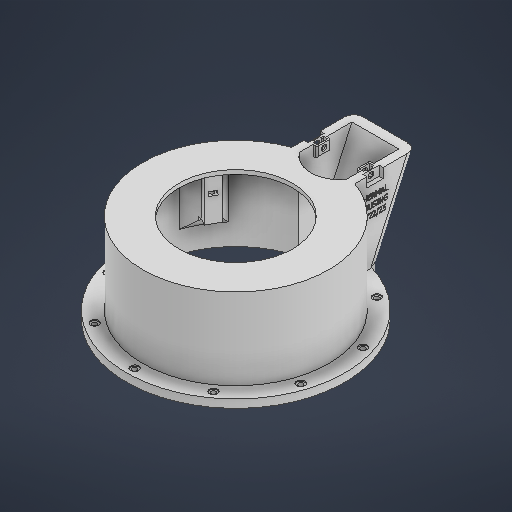
# Autodesk Inventor part: Thermal Housing
Saved by Autodesk Inventor 2026.2 (Build 302298000, 298)
## iProperties
Created: 2025-12-15
Part Number: Thermal Housing
Material: Generic
Document SubType Name: Modeling
Designer: mayhe
Density: 1 g/cm^3
Appearance: Default
Author: mayhe
Autodesk Inventor part; units mm, degrees
ref_plane "YZ Plane" through (0, 0, 0) normal (1, 0, 0) x (0, 1, 0)
ref_plane "XZ Plane" through (0, 0, 0) normal (0, 1, 0) x (-1, 0, 0)
ref_plane "XY Plane" through (0, 0, 0) normal (0, 0, 1) x (1, 0, 0)
sketch "Sketch1" plane through (0, 0, 0) normal (0, 1, 0) x (-1, 0, 0)
  circle A0 centre (0, 0) radius 135
  circle A1 centre (0, 0) radius 110.125
  circle A2 centre (0, 0) radius 115
  line L0 (39, -133.175) -> (-39, -133.175)
  line L1 (-39, -133.175) -> (-39, -87.525)
  line L2 (-39, -87.525) -> (39, -87.525)
  line L3 (39, -87.525) -> (39, -130.675)
  line L4 (39, -130.675) -> (39, -133.175)
  point P0 (0, -135)
  point P1 (39, -129.244)
  point P2 (-39, -129.244)
  point P3 (39, -130.675)
  point P4 (39, -102.9879)
  point P5 (39, -108.185)
  point P6 (-39, -108.185)
  point P7 (-39, -102.9879)
  dimension "d0" = 270
  dimension "d1" = 220.25
  dimension "d10" = 4.875
  dimension "d17" = 78
  dimension "d38" = 133.175
  dimension "d106" = 39
  dimension "d107" = 78
  constraints: 10 end point, 2 centre point, 2 coincident, 2 parallel, 1 horizontal, 1 perpendicular, 3 other
  measures "d1" diameter of A1
  measures "d10" radial gap between concentric circles of A1 A2
  measures "d17" distance of L1.end L2.end
  measures "d38" distance from line of A1.centre L0
  measures "d106" distance from line of point (0, 0) L1
  measures "d107" distance of L0.start L0.end
extrude "Cylinder Base" add sketch "Sketch1" along normal blind 10 contours A0 L3 A2 L1 | L1 A2 L3 A0 L0 | A0 L0 L1 | L3 L4 L0 A0 | L1 A1 L3 A2 | A2 L3 A1 L1
extrude "Cylinder Walls" add sketch "Sketch1" along normal blind 110.5 contours A2 L3 A1 L1 picked at (82.5972, -75.0251)
sketch "Sketch4" plane through (0, 110.5, 0) normal (0, 1, 0) x (1, 0, 0)
  circle A0 centre (0, 0) radius 110.125
  circle A1 centre (0, 0) radius 70.375
  dimension "d27" = 140.75
  constraints: 2 centre point, 2 coincident
  measures "d27" diameter of A1
extrude "Cylinder Top" add sketch "Sketch4" against normal blind 5
sketch "Sketch5" plane through (0, 110.5, 0) normal (0, 1, 0) x (1, 0, 0)
  line L0 (39, 108.185) -> (39, 185)
  line L1 (39, 185) -> (-39, 185)
  line L2 (-39, 185) -> (-39, 108.185)
  line L3 (-29, 172.6754) -> (29, 172.6754)
  line L4 (29, 172.6754) -> (29, 117.6754)
  line L5 (29, 117.6754) -> (-39, 117.6754)
  line L6 (-29, 117.6754) -> (-29, 172.6754)
  line L7 (-29, 172.6754) -> (29, 117.6754) construction
  line L8 (29, 172.6754) -> (-29, 117.6754) construction
  arc A0 (-29, 117.6754) -> (29, 117.6754) centre (0, 128.2867) ccw
  line L9 (39, 102.9879) -> (39, 108.185) projected
  line L10 (39, 108.185) -> (39, 102.9879)
  line L11 (-39, 108.185) -> (-39, 102.9879) projected
  line L12 (-39, 102.9879) -> (-39, 108.185)
  arc A1 (39, 102.9879) -> (-39, 102.9879) centre (0, 0) ccw projected
  line L13 (-39, 104.6754) -> (-39, 94.6754)
  line L14 (-39, 94.6754) -> (39, 94.6754)
  line L15 (39, 94.6754) -> (39, 102.9879)
  line L16 (29, 117.6754) -> (39, 117.6754)
  line L17 (-33.65, 177.3254) -> (33.65, 177.3254)
  line L18 (33.65, 177.3254) -> (33.65, 116.8811)
  arc A2 (-33.65, 116.8811) -> (33.65, 116.8811) centre (0, 128.2867) ccw
  line L19 (-33.65, 116.8811) -> (-33.65, 177.3254)
  line L20 (-29, 117.6754) -> (-29, 107.7584)
  line L21 (29, 117.6754) -> (29, 107.7584)
  point P0 (0, 113.425)
  point P1 (0, 145.1754)
  point P2 (23.0117, 107.6939)
  point P3 (-23.0117, 107.6939)
  point P4 (-39, 102.9879)
  point P5 (-39, 102.9879)
  point P6 (29, 106.238)
  point P7 (29, 106.4999)
  point P8 (-11.5192, 94.6754)
  point P9 (11.5192, 94.6754)
  point P10 (-33.65, 117.6754)
  point P11 (33.65, 117.6754)
  point P12 (-29, 106.238)
  point P13 (-28.0594, 106.4903)
  point P14 (28.0594, 106.4903)
  dimension "d33" = 78
  dimension "d36" = 55
  dimension "d72" = 185
  dimension "d115" = 10
  dimension "d132" = 78
  dimension "d133" = 10
  dimension "d134" = 23
  dimension "d135" = 4.65
  dimension "d150" = 10
  constraints: 40 end point, 7 point on circle, 4 point on line, 2 centre point, 2 midpoint, 2 parallel, 2 vertical, 1 perpendicular, 3 other
  measures "d33" distance between parallel lines of L2 L0
  measures "d36" distance of L3.end L4.end
  measures "d72" distance from line of point (0, 0) L1
  measures "d115" distance between parallel lines of L4 L0
  measures "d132" distance of L14.end L13.end
  measures "d133" distance of L13.end L13.start
  measures "d134" distance between parallel lines of L14 L5
  measures "d135" distance between parallel lines of L6 L19
  measures "d150" distance between parallel lines of L6 L2
sketch "Sketch6" plane through (0, 0, 0) normal (1, 0, 0) x (0, 1, 0)
  line L0 (110.5, -110.125) -> (110.5, -102.9879) projected
  line L1 (110.5, -178.433) -> (10, -133.175)
  line L2 (10, -133.175) -> (0, -133.175)
  point P0 (0, 0)
  point P1 (110.5, -108.185)
  dimension "d41" = 70.248
  constraints: 4 end point, 1 horizontal
  measures "d41" distance of point (110.5, -108.185) L1.start
sweep "Angled Camera Bracket" add profiles "Sketch5" path "Sketch6" keep normal constant yes path curves L1 L2 contours L9 A1 A2 L18 L16 L0 | L16 L18 L17 L19 L5 L2 L1 L0 | L18 A2 L21 L16 | L16 L4 L3 L6 L5 L19 L17 L18 | A1 A0 L21 A2 | L5 L19 A2 A1 L11 L2 | L20 A2 L19 L5 | A0 A1 A2 L20
extrude "Camera Clearance Cutout" cut sketch "Sketch5" against normal blind 25 contours A2 L14 A1 A0 | A1 A0 L21 A2 | A0 A1 L5 | A0 A1 | A2 L14 | A0 A1 A2 L20
sketch "Sketch7" plane through (0, 0, 0) normal (0, -1, 0) x (1, 0, 0)
  circle A0 centre (0, 0) radius 110.125
  constraints: 1 centre point, 1 coincident
extrude "Remove Excess from Sweep" cut sketch "Sketch7" against normal up to surface (105.5 mm away)
sketch "Sketch9" plane through (0, 0, 0) normal (1, 0, 0) x (0, 1, 0)
  point P0 (0, 0)
sketch "Sketch10" plane through (39, 110.5, -185) normal (0, -0.4106138, -0.9118093) x (-1, 0, 0)
  circle A0 centre (39, -58.2204) radius 3.5
  circle A1 centre (39, -44.2204) radius 3.5
  line L0 (78, 0) -> (78, -110.2204) projected
  line L1 (78, -110.2204) -> (0, -110.2204) projected
  point P0 (39, -176.7185)
  dimension "d61" = 7
  dimension "d63" = 7
  dimension "d64" = 14
  dimension "d108" = 39
  dimension "d168" = 52
  constraints: 2 centre point, 1 vertical alignment
  measures "d61" diameter of A0
  measures "d63" diameter of A1
  measures "d64" distance of A0.centre A1.centre
  measures "d108" distance from line of L0 A0.centre
  measures "d168" distance from line of L1 A0.centre
hole "Hole2" at (0, 70.1794, -166.8425) at (0, 57.4141, -161.0939) direction (0, 0.4106138, 0.9118093) diameter 7.25 depth 17.1 tip angle 118 counterbore diameter 12 counterbore depth 1.2
sketch "Sketch16" plane through (39, 0, -129.244) normal (1, 0, 0) x (0, 0, -1)
  line L0 (43.4315, 110.5) -> (-11.5685, 110.5) projected
  line L1 (-6.0589, 110.5) -> (13.9411, 110.5)
  line L2 (13.9411, 110.5) -> (13.9411, 98.5)
  line L3 (13.9411, 98.5) -> (-6.0589, 98.5)
  line L4 (-6.0589, 98.5) -> (-6.0589, 110.5)
  line L5 (-21.0589, 10) -> (-21.0589, 110.5) projected
  point P0 (-129.244, 0)
  point P1 (-22.7347, 10)
  dimension "d109" = 20
  dimension "d110" = 12
  dimension "d111" = 15
  constraints: 8 end point, 2 parallel, 1 horizontal, 1 perpendicular, 1 point on line, 1 other
  measures "d109" distance of L2.end L3.end
  measures "d110" distance of L1.end L2.end
extrude "Extrusion15" cut sketch "Sketch16" along normal through all both and the other way through all
sketch "Sketch17" plane through (39, 98.5, -123.185) normal (0, 1, 0) x (1, 0, 0)
  line L0 (-10, 0) -> (0, 0) projected
  line L1 (0, 20) -> (-10, 20) projected
  line L2 (-10, 0) -> (-5, 0)
  line L3 (-5, 0) -> (-5, 20)
  line L4 (-5, 20) -> (-7.675, 20)
  line L5 (-15, 1.5) -> (-10, 1.5)
  line L6 (-5, 3) -> (-5, 17)
  line L7 (-15, 18.5) -> (-15, 1.5)
  line L8 (-15, 1.5) -> (-5, 17) construction
  line L9 (-5, 3) -> (-15, 18.5) construction
  line L10 (-10, 1.5) -> (-10, 0)
  line L11 (-10, 0) -> (-10, 20) projected
  line L12 (-15, 18.5) -> (-10, 18.5)
  line L13 (-10, 18.5) -> (-10, 20)
  point P0 (-39, -123.185)
  point P1 (-5.35, 0)
  point P2 (-7.675, 20)
  dimension "d116" = 14
  dimension "d162" = 17
  dimension "d163" = 1.5
  constraints: 22 end point, 3 parallel, 3 perpendicular, 2 horizontal, 2 point on line, 1 collinear, 1 midpoint
  measures "d116" distance of L6.end L6.start
  measures "d162" distance of L7.start L5.start
  measures "d163" distance between parallel lines of L0 L5
extrude "Extrusion16" add sketch "Sketch17" along normal blind 12 and the other way blind 1
sketch "Sketch18" plane through (0, 110.5, 0) normal (0, 1, 0) x (1, 0, 0)
  line L0 (26, 126.685) -> (31.15, 126.685)
  line L1 (31.15, 126.685) -> (31.15, 139.685)
  line L2 (31.15, 139.685) -> (26, 139.685)
  line L3 (26, 139.685) -> (26, 126.685)
  line L4 (26, 126.685) -> (31.15, 139.685) construction
  line L5 (31.15, 126.685) -> (26, 139.685) construction
  line L6 (24, 141.685) -> (24, 124.685) projected
  line L7 (29, 141.685) -> (24, 141.685) projected
  point P0 (0, 0)
  point P1 (28.575, 133.185)
  dimension "d121" = 5.15
  dimension "d122" = 13
  dimension "d123" = 2
  dimension "d160" = 2
  constraints: 12 end point, 2 midpoint, 2 parallel, 1 horizontal, 1 perpendicular
  measures "d121" distance of L2.end L1.end
  measures "d122" distance of L1.end L0.end
  measures "d123" distance between parallel lines of L6 L3
  measures "d160" distance between parallel lines of L7 L2
extrude "Extrusion17" cut sketch "Sketch18" against normal blind 11
sketch "Sketch19" plane through (34, 98.5, -123.185) normal (1, 0, 0) x (0, 0, -1)
  circle A0 centre (10, 6.5) radius 3.575
  line L0 (0, 12) -> (20, 12) projected
  line L1 (20, 12) -> (20, 0) projected
  point P0 (-123.185, -98.5)
  dimension "d126" = 7.15
  dimension "d127" = 5.5
  dimension "d128" = 10
  constraints: 1 centre point
  measures "d126" diameter of A0
  measures "d127" distance from line of L0 A0.centre
  measures "d128" distance from line of L1 A0.centre
extrude "Extrusion18" cut sketch "Sketch19" against normal blind 11
fillet "Fillet1" radius 2 3 edges at (24, 104, -124.685) (24, 97.5, -133.185) (24, 104, -141.685)
mirror "Mirror1" about plane through (0, 0, 0) normal (1, 0, 0) of "Extrusion16", "Extrusion18", "Extrusion17", "Fillet1"
sketch "Sketch20" plane through (0, 10, 0) normal (0, 1, 0) x (1, 0, 0)
  circle A0 centre (0, 0) radius 125
  circle A1 centre (0, -125) radius 2.5
  circle A2 centre (73.4732, -101.1271) radius 2.5
  circle A3 centre (118.8821, -38.6271) radius 2.5
  circle A4 centre (118.8821, 38.6271) radius 2.5
  circle A5 centre (73.4732, 101.1271) radius 2.5
  circle A6 centre (0, 125) radius 2.5
  circle A7 centre (-73.4732, 101.1271) radius 2.5
  circle A8 centre (-118.8821, 38.6271) radius 2.5
  circle A9 centre (-118.8821, -38.6271) radius 2.5
  circle A10 centre (-73.4732, -101.1271) radius 2.5
  dimension "d136" = 250
  dimension "d137" = 5
  dimension "d140" = 360
  constraints: 10 centre point, 1 coincident, 1 vertical alignment, 23 other
  measures "d137" diameter of A1
hole "Hole3" at (118.8821, 10, -38.6271) at (73.4732, 10, -101.1271) at (118.8821, 10, 38.6271) at (73.4732, 10, 101.1271) at (0, 10, 125) at (-73.4732, 10, 101.1271) at (-118.8821, 10, 38.6271) at (-118.8821, 10, -38.6271) at (-73.4732, 10, -101.1271) direction (0, -1, 0) diameter 5.9 depth 17.1 tip angle 118 counterbore diameter 10.2 counterbore depth 1.2
sketch "Sketch24" plane through (31.15, 110.5, -139.685) normal (-1, 0, 0) x (0, 0, 1)
  circle A0 centre (6.5, -5.5) radius 3.575 projected
  circle A1 centre (6.5, -5.5) radius 6.5
  point P0 (139.685, -110.5)
  dimension "d161" = 13
  constraints: 1 centre point, 1 coincident
  measures "d161" diameter of A1
extrude "Extrusion22" cut sketch "Sketch24" along normal blind 2 and the other way blind 1.9
mirror "Mirror2" about plane through (0, 0, 0) normal (1, 0, 0) of "Extrusion22"
fillet "Fillet3" radius 11 4 edges at (-39, 60.25, -162.371) (-39, 5, -139.742) (39, 60.25, -162.371) (39, 5, -139.742)
sketch "Sketch25" plane through (0, 105.5, 0) normal (0, -1, 0) x (1, 0, 0)
  line L0 (0, 0) -> (0, 150.8979)
  line L1 (0, 76) -> (8, 76)
  line L2 (8, 76) -> (8, 86)
  line L3 (0, 86) -> (0, 76)
  circle A0 centre (0, 0) radius 110.125
  line L4 (8, 86) -> (22.0087, 107.9034)
  arc A1 (39, -102.9879) -> (-39, -102.9879) centre (0, 0) ccw projected
  line L5 (0, 76) -> (-8, 76)
  line L6 (-8, 76) -> (-8, 86)
  line L7 (-8, 86) -> (-22.0087, 107.9034)
  point P0 (-28.0594, -106.4903)
  point P1 (28.0594, -106.4903)
  point P2 (22.0087, 107.9034)
  dimension "d177" = 26
  dimension "d178" = 10
  dimension "d179" = 8
  constraints: 16 end point, 3 symmetric about line, 1 centre point, 1 coincident, 1 horizontal, 1 parallel, 1 perpendicular, 1 point on circle, 1 point on line, 1 vertical
  measures "d177" distance of L2.end L4.end
  measures "d178" distance of L1.end L2.end
  measures "d179" distance of L1.start L1.end
extrude "HorseShoe Mount Body" add sketch "Sketch25" along normal blind 55 contours L5 L6 L7 A0 L0 | L0 A0 L4 L2 L1
sketch "Sketch26" plane through (0, 50.5, 0) normal (0, -1, 0) x (1, 0, 0)
  line L0 (0, -249) -> (0, 199) projected
  point P0 (0, 0)
  point P1 (0, 81)
  dimension "d192" = 81
  constraints: 1 point on line
  measures "d192" distance of point (0, 81) point (0, 0)
hole "Hole4" at (0, 50.5, 81) direction (0, 1, 0) diameter 5.2 depth 35
chamfer "Chamfer1" distance 24 angle 45 1 edges at (0, 50.5, 110.125)
sketch "Sketch27" plane through (0, 50.5, 0) normal (0, -1, 0) x (1, 0, 0)
  arc A0 (13.159, 89.0328) -> (-13.297, 89.0123) centre (0, 0) ccw
  line L0 (-22.0087, 107.9034) -> (-8, 86) projected
  line L1 (8, 86) -> (22.0087, 107.9034) projected
  line L2 (-13.297, 89.0123) -> (0, 0)
  line L3 (0, 0) -> (13.159, 89.0328)
  dimension "d193" = 90
  constraints: 4 end point, 2 point on circle, 1 centre point, 1 coincident
  measures "d193" radius of A0
extrude "HorseShoe Piece Cutout" cut sketch "Sketch27" along normal through all
ref_plane "Work Plane2" through (0, 81.5, 0) normal (0, -1, 0) x (1, 0, 0)
sketch "Sketch28" plane through (0, 81.5, 0) normal (0, -1, 0) x (1, 0, 0)
  circle A0 centre (0, 81) radius 2.6 projected
  line L0 (0, 85.5611) -> (3.95, 83.2805)
  line L1 (3.95, 83.2805) -> (3.95, 78.7195)
  line L2 (-3.95, 78.7195) -> (-3.95, 83.2805)
  line L3 (-3.95, 83.2805) -> (0, 85.5611)
  line L4 (8, 76) -> (-8, 76) projected
  line L5 (3.95, 78.7195) -> (3.95, 76)
  line L6 (3.95, 76) -> (-3.95, 76)
  line L7 (-3.95, 76) -> (-3.95, 78.7195)
  point P0 (0, 0)
  point P1 (-3.95, 76)
  dimension "d197" = 7.9
  constraints: 14 end point, 1 coincident, 1 parallel, 1 point on line, 8 other
  measures "d197" distance between parallel lines of L1 L2
extrude "Nut Seat" cut sketch "Sketch28" against normal blind 4 contours A0 | L0 L1 L5 L4 L7 L2 L3
sketch "Sketch29" plane through (0, 81.5, 0) normal (0, -1, 0) x (1, 0, 0)
  circle A0 centre (0, 81) radius 2.6 projected
  arc A1 (4.5, 81) -> (-4.5, 81) centre (0, 81) ccw
  line L0 (8, 76) -> (-8, 76) projected
  line L1 (4.5, 81) -> (4.5, 76)
  line L2 (4.5, 76) -> (-4.5, 76)
  line L3 (-4.5, 76) -> (-4.5, 81)
  point P0 (0, 0)
  dimension "d200" = 9
  constraints: 6 end point, 2 point on circle, 1 centre point, 1 coincident, 1 parallel, 1 point on line
  measures "d200" diameter of A1
extrude "Washer Seat" cut sketch "Sketch29" along normal blind 1.1 contours A0 | L1 L0 L3 A1
chamfer "Washer Insert Chamfer" distance 0.5 angle 45 4 edges at (-3.95, 81.5, 79.5779) (-1.975, 81.5, 84.4208) (1.975, 81.5, 84.4208) (3.95, 81.5, 79.5779)
pattern_circular "Circular Pattern2" count 3 over 360 about axis through (0, 0, 0) along (0, 1, 0) of "HorseShoe Mount Body", "Hole4", "Chamfer1", "HorseShoe Piece Cutout", "Nut Seat", "Washer Seat"
sketch "Sketch30" plane through (39, 10, -108.185) normal (1, 0, 0) x (0, 0, -1)
  line L0 (5.006, 79.9076) -> (42.4169, 79.9076) construction
  line L1 (42.4169, 79.9076) -> (42.4169, 71.115) construction
  line L2 (42.4169, 71.115) -> (5.006, 71.115) construction
  line L3 (5.006, 71.115) -> (5.006, 79.9076) construction
  line L4 (7.0463, 73.8116) -> (7.0463, 79.1864)
  line L5 (7.0463, 79.1864) -> (5.0011, 79.1864)
  line L6 (5.0011, 79.1864) -> (5.0011, 79.9076)
  line L7 (5.0011, 79.9076) -> (9.9016, 79.9076)
  line L8 (9.9016, 79.9076) -> (9.9016, 79.1864)
  line L9 (9.9016, 79.1864) -> (7.8564, 79.1864)
  line L10 (7.8564, 79.1864) -> (7.8564, 73.8116)
  line L11 (7.8564, 73.8116) -> (7.0463, 73.8116)
  line L12 (14.9454, 73.8116) -> (14.1352, 73.8116)
  line L13 (14.1352, 73.8116) -> (14.1352, 76.7954)
  line L14 (14.1352, 76.7954) -> (11.3293, 76.7954)
  line L15 (11.3293, 76.7954) -> (11.3293, 73.8116)
  line L16 (11.3293, 73.8116) -> (10.5191, 73.8116)
  line L17 (10.5191, 73.8116) -> (10.5191, 79.9076)
  line L18 (10.5191, 79.9076) -> (11.3293, 79.9076)
  line L19 (11.3293, 79.9076) -> (11.3293, 77.5166)
  line L20 (11.3293, 77.5166) -> (14.1352, 77.5166)
  line L21 (14.1352, 77.5166) -> (14.1352, 79.9076)
  line L22 (14.1352, 79.9076) -> (14.9454, 79.9076)
  line L23 (14.9454, 79.9076) -> (14.9454, 73.8116)
  line L24 (16.1804, 73.8116) -> (16.1804, 79.9076)
  line L25 (16.1804, 79.9076) -> (19.9941, 79.9076)
  line L26 (19.9941, 79.9076) -> (19.9941, 79.1864)
  line L27 (19.9941, 79.1864) -> (16.9906, 79.1864)
  line L28 (16.9906, 79.1864) -> (16.9906, 77.5166)
  line L29 (16.9906, 77.5166) -> (19.7916, 77.5166)
  line L30 (19.7916, 77.5166) -> (19.7916, 76.7954)
  line L31 (19.7916, 76.7954) -> (16.9906, 76.7954)
  line L32 (16.9906, 76.7954) -> (16.9906, 74.5329)
  line L33 (16.9906, 74.5329) -> (19.9941, 74.5329)
  line L34 (19.9941, 74.5329) -> (19.9941, 73.8116)
  line L35 (19.9941, 73.8116) -> (16.1804, 73.8116)
  line L36 (25.601, 73.8116) -> (24.5488, 73.8116)
  line L37 (24.5488, 73.8116) -> (22.6222, 76.2372)
  line L38 (22.6222, 76.2372) -> (21.6935, 76.2372)
  line L39 (21.6935, 76.2372) -> (21.6935, 73.8116)
  line L40 (21.6935, 73.8116) -> (20.8833, 73.8116)
  line L41 (20.8833, 73.8116) -> (20.8833, 79.9076)
  line L42 (20.8833, 79.9076) -> (22.4542, 79.9076)
  spline S0 degree 2 poles (22.4542, 79.9076) (22.9779, 79.9076) (23.6843, 79.794) (24.0054, 79.5865) knots 0 0 0 1 2 2 2
  spline S1 degree 2 poles (24.0054, 79.5865) (24.3265, 79.379) (24.697, 78.7319) (24.697, 78.2527) knots 0 0 0 1 2 2 2
  spline S2 degree 2 poles (24.697, 78.2527) (24.697, 77.5858) (24.0153, 76.6818) (23.4324, 76.4644) knots 0 0 0 1 2 2 2
  line L43 (23.4324, 76.4644) -> (25.601, 73.8116)
  spline S3 degree 2 poles (23.8523, 78.1885) (23.8523, 78.4553) (23.6645, 78.8653) (23.4669, 78.9987) knots 0 0 0 1 2 2 2
  spline S4 degree 2 poles (23.4669, 78.9987) (23.294, 79.1123) (22.8346, 79.2061) (22.4987, 79.2061) knots 0 0 0 1 2 2 2
  line L44 (22.4987, 79.2061) -> (21.6935, 79.2061)
  line L45 (21.6935, 79.2061) -> (21.6935, 76.914)
  line L46 (21.6935, 76.914) -> (22.4048, 76.914)
  spline S5 degree 2 poles (22.4048, 76.914) (22.7556, 76.914) (23.3138, 77.0375) (23.5065, 77.2301) knots 0 0 0 1 2 2 2
  spline S6 degree 2 poles (23.5065, 77.2301) (23.6843, 77.3981) (23.8523, 77.8723) (23.8523, 78.1885) knots 0 0 0 1 2 2 2
  line L47 (31.3117, 73.8116) -> (30.5016, 73.8116)
  line L48 (30.5016, 73.8116) -> (30.5016, 79.0629)
  line L49 (30.5016, 79.0629) -> (28.9109, 75.4912)
  line L50 (28.9109, 75.4912) -> (28.4169, 75.4912)
  line L51 (28.4169, 75.4912) -> (26.841, 79.0629)
  line L52 (26.841, 79.0629) -> (26.841, 73.8116)
  line L53 (26.841, 73.8116) -> (26.0852, 73.8116)
  line L54 (26.0852, 73.8116) -> (26.0852, 79.9076)
  line L55 (26.0852, 79.9076) -> (27.1917, 79.9076)
  line L56 (27.1917, 79.9076) -> (28.7133, 76.5138)
  line L57 (28.7133, 76.5138) -> (30.1854, 79.9076)
  line L58 (30.1854, 79.9076) -> (31.3117, 79.9076)
  line L59 (31.3117, 79.9076) -> (31.3117, 73.8116)
  line L60 (31.8897, 73.8116) -> (33.9448, 79.9076)
  line L61 (33.9448, 79.9076) -> (34.9426, 79.9076)
  line L62 (34.9426, 79.9076) -> (36.9977, 73.8116)
  line L63 (36.9977, 73.8116) -> (36.1431, 73.8116)
  line L64 (36.1431, 73.8116) -> (35.5898, 75.5159)
  line L65 (35.5898, 75.5159) -> (33.263, 75.5159)
  line L66 (33.263, 75.5159) -> (32.7097, 73.8116)
  line L67 (32.7097, 73.8116) -> (31.8897, 73.8116)
  line L68 (35.3675, 76.2075) -> (34.4239, 79.0777)
  line L69 (34.4239, 79.0777) -> (33.4853, 76.2075)
  line L70 (33.4853, 76.2075) -> (35.3675, 76.2075)
  line L71 (41.1078, 73.8116) -> (37.5757, 73.8116)
  line L72 (37.5757, 73.8116) -> (37.5757, 79.9076)
  line L73 (37.5757, 79.9076) -> (38.3858, 79.9076)
  line L74 (38.3858, 79.9076) -> (38.3858, 74.5329)
  line L75 (38.3858, 74.5329) -> (41.1078, 74.5329)
  line L76 (41.1078, 74.5329) -> (41.1078, 73.8116)
  line L77 (10.0498, 63.7747) -> (9.2397, 63.7747)
  line L78 (9.2397, 63.7747) -> (9.2397, 66.7585)
  line L79 (9.2397, 66.7585) -> (6.4337, 66.7585)
  line L80 (6.4337, 66.7585) -> (6.4337, 63.7747)
  line L81 (6.4337, 63.7747) -> (5.6235, 63.7747)
  line L82 (5.6235, 63.7747) -> (5.6235, 69.8707)
  line L83 (5.6235, 69.8707) -> (6.4337, 69.8707)
  line L84 (6.4337, 69.8707) -> (6.4337, 67.4797)
  line L85 (6.4337, 67.4797) -> (9.2397, 67.4797)
  line L86 (9.2397, 67.4797) -> (9.2397, 69.8707)
  line L87 (9.2397, 69.8707) -> (10.0498, 69.8707)
  line L88 (10.0498, 69.8707) -> (10.0498, 63.7747)
  spline S7 degree 2 poles (15.5975, 69.1742) (15.9433, 68.7691) (16.3286, 67.5835) (16.3286, 66.8227) knots 0 0 0 1 2 2 2
  spline S8 degree 2 poles (16.3286, 66.8227) (16.3286, 66.0817) (15.9532, 64.8813) (15.5975, 64.4762) knots 0 0 0 1 2 2 2
  spline S9 degree 2 poles (15.5975, 64.4762) (15.222, 64.0514) (14.2291, 63.6463) (13.6313, 63.6463) knots 0 0 0 1 2 2 2
  spline S10 degree 2 poles (13.6313, 63.6463) (13.0138, 63.6463) (12.0258, 64.0662) (11.6652, 64.4762) knots 0 0 0 1 2 2 2
  spline S11 degree 2 poles (11.6652, 64.4762) (11.3145, 64.8813) (10.939, 66.0718) (10.939, 66.8227) knots 0 0 0 1 2 2 2
  spline S12 degree 2 poles (10.939, 66.8227) (10.939, 67.5884) (11.3194, 68.7543) (11.6701, 69.1742) knots 0 0 0 1 2 2 2
  spline S13 degree 2 poles (11.6701, 69.1742) (12.0258, 69.5793) (13.0188, 69.9992) (13.6313, 69.9992) knots 0 0 0 1 2 2 2
  spline S14 degree 2 poles (13.6313, 69.9992) (14.2538, 69.9992) (15.2517, 69.5644) (15.5975, 69.1742) knots 0 0 0 1 2 2 2
  spline S15 degree 2 poles (15.4839, 66.8227) (15.4839, 67.4254) (15.222, 68.3591) (14.9849, 68.6654) knots 0 0 0 1 2 2 2
  spline S16 degree 2 poles (14.9849, 68.6654) (14.7428, 68.9815) (14.0611, 69.2977) (13.6363, 69.2977) knots 0 0 0 1 2 2 2
  spline S17 degree 2 poles (13.6363, 69.2977) (13.1966, 69.2977) (12.5347, 68.9914) (12.2827, 68.6654) knots 0 0 0 1 2 2 2
  spline S18 degree 2 poles (12.2827, 68.6654) (12.0406, 68.3541) (11.7838, 67.4155) (11.7838, 66.8227) knots 0 0 0 1 2 2 2
  spline S19 degree 2 poles (11.7838, 66.8227) (11.7838, 65.6223) (12.7915, 64.3478) (13.6363, 64.3478) knots 0 0 0 1 2 2 2
  spline S20 degree 2 poles (13.6363, 64.3478) (14.481, 64.3478) (15.4839, 65.6223) (15.4839, 66.8227) knots 0 0 0 1 2 2 2
  spline S21 degree 2 poles (19.347, 63.6463) (18.8085, 63.6463) (18.0082, 63.9279) (17.7266, 64.2094) knots 0 0 0 1 2 2 2
  spline S22 degree 2 poles (17.7266, 64.2094) (17.4055, 64.5256) (17.1437, 65.4148) (17.1437, 66.0669) knots 0 0 0 1 2 2 2
  line L89 (17.1437, 66.0669) -> (17.1437, 69.8707)
  line L90 (17.1437, 69.8707) -> (17.9539, 69.8707)
  line L91 (17.9539, 69.8707) -> (17.9539, 66.0669)
  spline S23 degree 2 poles (17.9539, 66.0669) (17.9539, 65.6421) (18.0625, 65.069) (18.2157, 64.8368) knots 0 0 0 1 2 2 2
  spline S24 degree 2 poles (18.2157, 64.8368) (18.3787, 64.5898) (18.9419, 64.3379) (19.347, 64.3379) knots 0 0 0 1 2 2 2
  spline S25 degree 2 poles (19.347, 64.3379) (19.7273, 64.3379) (20.3201, 64.5898) (20.4832, 64.8368) knots 0 0 0 1 2 2 2
  spline S26 degree 2 poles (20.4832, 64.8368) (20.6363, 65.069) (20.745, 65.6371) (20.745, 66.0471) knots 0 0 0 1 2 2 2
  line L92 (20.745, 66.0471) -> (20.745, 69.8707)
  line L93 (20.745, 69.8707) -> (21.5552, 69.8707)
  line L94 (21.5552, 69.8707) -> (21.5552, 66.0669)
  spline S27 degree 2 poles (21.5552, 66.0669) (21.5552, 65.4296) (21.2983, 64.5207) (20.9722, 64.2094) knots 0 0 0 1 2 2 2
  spline S28 degree 2 poles (20.9722, 64.2094) (20.6808, 63.9229) (19.9101, 63.6463) (19.347, 63.6463) knots 0 0 0 1 2 2 2
  spline S29 degree 2 poles (24.4154, 63.666) (23.7535, 63.666) (22.8247, 63.9427) (22.4147, 64.1403) knots 0 0 0 1 2 2 2
  line L95 (22.4147, 64.1403) -> (22.4147, 65.1579)
  line L96 (22.4147, 65.1579) -> (22.474, 65.1579)
  spline S30 degree 2 poles (22.474, 65.1579) (22.8741, 64.7825) (23.8868, 64.3675) (24.3561, 64.3675) knots 0 0 0 1 2 2 2
  spline S31 degree 2 poles (24.3561, 64.3675) (25.028, 64.3675) (25.7147, 64.9257) (25.7147, 65.3852) knots 0 0 0 1 2 2 2
  spline S32 degree 2 poles (25.7147, 65.3852) (25.7147, 65.7507) (25.354, 66.2052) (24.9638, 66.3188) knots 0 0 0 1 2 2 2
  spline S33 degree 2 poles (24.9638, 66.3188) (24.6822, 66.3979) (24.2129, 66.5066) (23.8621, 66.5955) knots 0 0 0 1 2 2 2
  spline S34 degree 2 poles (23.8621, 66.5955) (23.546, 66.6795) (23.047, 66.9314) (22.8544, 67.1339) knots 0 0 0 1 2 2 2
  spline S35 degree 2 poles (22.8544, 67.1339) (22.6667, 67.3365) (22.4592, 67.8799) (22.4592, 68.2356) knots 0 0 0 1 2 2 2
  spline S36 degree 2 poles (22.4592, 68.2356) (22.4592, 68.9766) (23.6151, 69.9794) (24.5093, 69.9794) knots 0 0 0 1 2 2 2
  spline S37 degree 2 poles (24.5093, 69.9794) (25.0231, 69.9794) (25.932, 69.7769) (26.3223, 69.5842) knots 0 0 0 1 2 2 2
  line L97 (26.3223, 69.5842) -> (26.3223, 68.616)
  line L98 (26.3223, 68.616) -> (26.263, 68.616)
  spline S38 degree 2 poles (26.263, 68.616) (25.9715, 68.8827) (25.0626, 69.2779) (24.5636, 69.2779) knots 0 0 0 1 2 2 2
  spline S39 degree 2 poles (24.5636, 69.2779) (24.0005, 69.2779) (23.3039, 68.7493) (23.3039, 68.3195) knots 0 0 0 1 2 2 2
  spline S40 degree 2 poles (23.3039, 68.3195) (23.3039, 67.9342) (23.7139, 67.4748) (24.0993, 67.3711) knots 0 0 0 1 2 2 2
  spline S41 degree 2 poles (24.0993, 67.3711) (24.3561, 67.3019) (25.1021, 67.1241) (25.3491, 67.05) knots 0 0 0 1 2 2 2
  spline S42 degree 2 poles (25.3491, 67.05) (25.9765, 66.8573) (26.5594, 66.0817) (26.5594, 65.5136) knots 0 0 0 1 2 2 2
  spline S43 degree 2 poles (26.5594, 65.5136) (26.5594, 65.153) (26.2679, 64.4614) (26.0061, 64.2193) knots 0 0 0 1 2 2 2
  spline S44 degree 2 poles (26.0061, 64.2193) (25.7147, 63.9526) (24.9737, 63.666) (24.4154, 63.666) knots 0 0 0 1 2 2 2
  line L99 (29.5086, 63.7747) -> (27.1473, 63.7747)
  line L100 (27.1473, 63.7747) -> (27.1473, 64.3972)
  line L101 (27.1473, 64.3972) -> (27.9229, 64.3972)
  line L102 (27.9229, 64.3972) -> (27.9229, 69.2483)
  line L103 (27.9229, 69.2483) -> (27.1473, 69.2483)
  line L104 (27.1473, 69.2483) -> (27.1473, 69.8707)
  line L105 (27.1473, 69.8707) -> (29.5086, 69.8707)
  line L106 (29.5086, 69.8707) -> (29.5086, 69.2483)
  line L107 (29.5086, 69.2483) -> (28.733, 69.2483)
  line L108 (28.733, 69.2483) -> (28.733, 64.3972)
  line L109 (28.733, 64.3972) -> (29.5086, 64.3972)
  line L110 (29.5086, 64.3972) -> (29.5086, 63.7747)
  line L111 (34.8735, 63.7747) -> (33.9645, 63.7747)
  line L112 (33.9645, 63.7747) -> (31.2673, 69.0309)
  line L113 (31.2673, 69.0309) -> (31.2673, 63.7747)
  line L114 (31.2673, 63.7747) -> (30.5114, 63.7747)
  line L115 (30.5114, 63.7747) -> (30.5114, 69.8707)
  line L116 (30.5114, 69.8707) -> (31.6625, 69.8707)
  line L117 (31.6625, 69.8707) -> (34.1177, 65.0443)
  line L118 (34.1177, 65.0443) -> (34.1177, 69.8707)
  line L119 (34.1177, 69.8707) -> (34.8735, 69.8707)
  line L120 (34.8735, 69.8707) -> (34.8735, 63.7747)
  spline S45 degree 2 poles (38.6625, 63.6562) (38.0153, 63.6562) (36.9434, 64.0514) (36.558, 64.4515) knots 0 0 0 1 2 2 2
  spline S46 degree 2 poles (36.558, 64.4515) (36.1727, 64.8566) (35.7627, 66.0521) (35.7627, 66.8277) knots 0 0 0 1 2 2 2
  spline S47 degree 2 poles (35.7627, 66.8277) (35.7627, 67.5637) (36.1776, 68.7296) (36.563, 69.1445) knots 0 0 0 1 2 2 2
  spline S48 degree 2 poles (36.563, 69.1445) (36.9335, 69.5447) (38.0203, 69.9794) (38.6674, 69.9794) knots 0 0 0 1 2 2 2
  spline S49 degree 2 poles (38.6674, 69.9794) (38.9786, 69.9794) (39.5418, 69.8905) (39.7987, 69.8114) knots 0 0 0 1 2 2 2
  spline S50 degree 2 poles (39.7987, 69.8114) (40.0062, 69.7522) (40.5101, 69.5348) (40.6632, 69.4558) knots 0 0 0 1 2 2 2
  line L121 (40.6632, 69.4558) -> (40.6632, 68.4776)
  line L122 (40.6632, 68.4776) -> (40.594, 68.4776)
  spline S51 degree 2 poles (40.594, 68.4776) (40.4409, 68.611) (40.1198, 68.8531) (39.8234, 68.9914) knots 0 0 0 1 2 2 2
  spline S52 degree 2 poles (39.8234, 68.9914) (39.5764, 69.1149) (38.9391, 69.2779) (38.5736, 69.2779) knots 0 0 0 1 2 2 2
  spline S53 degree 2 poles (38.5736, 69.2779) (37.6942, 69.2779) (36.6074, 67.954) (36.6074, 66.8524) knots 0 0 0 1 2 2 2
  spline S54 degree 2 poles (36.6074, 66.8524) (36.6074, 66.2398) (36.894, 65.3209) (37.1657, 65.0048) knots 0 0 0 1 2 2 2
  spline S55 degree 2 poles (37.1657, 65.0048) (37.4275, 64.6886) (38.1685, 64.3576) (38.6328, 64.3576) knots 0 0 0 1 2 2 2
  spline S56 degree 2 poles (38.6328, 64.3576) (38.9737, 64.3576) (39.6554, 64.4564) (39.8876, 64.5552) knots 0 0 0 1 2 2 2
  line L123 (39.8876, 64.5552) -> (39.8876, 66.1311)
  line L124 (39.8876, 66.1311) -> (38.4748, 66.1311)
  line L125 (38.4748, 66.1311) -> (38.4748, 66.8425)
  line L126 (38.4748, 66.8425) -> (40.6879, 66.8425)
  line L127 (40.6879, 66.8425) -> (40.6879, 64.1798)
  spline S57 degree 2 poles (40.6879, 64.1798) (40.5348, 64.1106) (40.0111, 63.8982) (39.7888, 63.834) knots 0 0 0 1 2 2 2
  spline S58 degree 2 poles (39.7888, 63.834) (39.4875, 63.7451) (39.0033, 63.6562) (38.6625, 63.6562) knots 0 0 0 1 2 2 2
  line L128 (8.9037, 53.7378) -> (5.9298, 53.7378)
  line L129 (5.9298, 53.7378) -> (5.9298, 54.3603)
  line L130 (5.9298, 54.3603) -> (7.0364, 54.3603)
  line L131 (7.0364, 54.3603) -> (7.0364, 58.4457)
  line L132 (7.0364, 58.4457) -> (5.9298, 58.4457)
  line L133 (5.9298, 58.4457) -> (5.9298, 59.0039)
  spline S59 degree 2 poles (5.9298, 59.0039) (6.5572, 59.0039) (7.15, 59.3596) (7.1895, 59.8536) knots 0 0 0 1 2 2 2
  line L134 (7.1895, 59.8536) -> (7.8219, 59.8536)
  line L135 (7.8219, 59.8536) -> (7.8219, 54.3603)
  line L136 (7.8219, 54.3603) -> (8.9037, 54.3603)
  line L137 (8.9037, 54.3603) -> (8.9037, 53.7378)
  line L138 (13.7845, 53.7378) -> (10.0251, 53.7378)
  line L139 (10.0251, 53.7378) -> (10.0251, 54.6023)
  spline S60 degree 2 poles (10.0251, 54.6023) (10.4302, 54.9827) (11.1514, 55.6891) (11.4972, 56.0695) knots 0 0 0 1 2 2 2
  spline S61 degree 2 poles (11.4972, 56.0695) (12.1938, 56.8352) (12.7026, 57.7541) (12.7026, 58.2431) knots 0 0 0 1 2 2 2
  spline S62 degree 2 poles (12.7026, 58.2431) (12.7026, 58.5) (12.5445, 58.8853) (12.4013, 59.0088) knots 0 0 0 1 2 2 2
  spline S63 degree 2 poles (12.4013, 59.0088) (12.258, 59.1323) (11.8826, 59.2558) (11.6553, 59.2558) knots 0 0 0 1 2 2 2
  spline S64 degree 2 poles (11.6553, 59.2558) (11.438, 59.2558) (10.9934, 59.1472) (10.7908, 59.0632) knots 0 0 0 1 2 2 2
  spline S65 degree 2 poles (10.7908, 59.0632) (10.6179, 58.994) (10.2968, 58.7964) (10.198, 58.7272) knots 0 0 0 1 2 2 2
  line L140 (10.198, 58.7272) -> (10.1536, 58.7272)
  line L141 (10.1536, 58.7272) -> (10.1536, 59.5967)
  spline S66 degree 2 poles (10.1536, 59.5967) (10.4055, 59.7202) (11.3095, 59.9623) (11.7146, 59.9623) knots 0 0 0 1 2 2 2
  spline S67 degree 2 poles (11.7146, 59.9623) (12.5692, 59.9623) (13.5325, 59.0582) (13.5325, 58.2876) knots 0 0 0 1 2 2 2
  spline S68 degree 2 poles (13.5325, 58.2876) (13.5325, 57.927) (13.3646, 57.3243) (13.2164, 57.0674) knots 0 0 0 1 2 2 2
  spline S69 degree 2 poles (13.2164, 57.0674) (13.0682, 56.8006) (12.6384, 56.277) (12.4013, 56.0251) knots 0 0 0 1 2 2 2
  spline S70 degree 2 poles (12.4013, 56.0251) (12.0159, 55.6051) (11.0724, 54.7061) (10.7908, 54.4442) knots 0 0 0 1 2 2 2
  line L142 (10.7908, 54.4442) -> (13.7845, 54.4442)
  line L143 (13.7845, 54.4442) -> (13.7845, 53.7378)
  line L144 (17.1338, 60.1055) -> (14.7478, 52.4139)
  line L145 (14.7478, 52.4139) -> (14.0562, 52.4139)
  line L146 (14.0562, 52.4139) -> (16.4323, 60.1055)
  line L147 (16.4323, 60.1055) -> (17.1338, 60.1055)
  line L148 (21.565, 53.7378) -> (17.8057, 53.7378)
  line L149 (17.8057, 53.7378) -> (17.8057, 54.6023)
  spline S71 degree 2 poles (17.8057, 54.6023) (18.2107, 54.9827) (18.932, 55.6891) (19.2778, 56.0695) knots 0 0 0 1 2 2 2
  spline S72 degree 2 poles (19.2778, 56.0695) (19.9743, 56.8352) (20.4832, 57.7541) (20.4832, 58.2431) knots 0 0 0 1 2 2 2
  spline S73 degree 2 poles (20.4832, 58.2431) (20.4832, 58.5) (20.3251, 58.8853) (20.1818, 59.0088) knots 0 0 0 1 2 2 2
  spline S74 degree 2 poles (20.1818, 59.0088) (20.0386, 59.1323) (19.6631, 59.2558) (19.4359, 59.2558) knots 0 0 0 1 2 2 2
  spline S75 degree 2 poles (19.4359, 59.2558) (19.2185, 59.2558) (18.7739, 59.1472) (18.5714, 59.0632) knots 0 0 0 1 2 2 2
  spline S76 degree 2 poles (18.5714, 59.0632) (18.3985, 58.994) (18.0774, 58.7964) (17.9786, 58.7272) knots 0 0 0 1 2 2 2
  line L150 (17.9786, 58.7272) -> (17.9341, 58.7272)
  line L151 (17.9341, 58.7272) -> (17.9341, 59.5967)
  spline S77 degree 2 poles (17.9341, 59.5967) (18.186, 59.7202) (19.0901, 59.9623) (19.4952, 59.9623) knots 0 0 0 1 2 2 2
  spline S78 degree 2 poles (19.4952, 59.9623) (20.3498, 59.9623) (21.3131, 59.0582) (21.3131, 58.2876) knots 0 0 0 1 2 2 2
  spline S79 degree 2 poles (21.3131, 58.2876) (21.3131, 57.927) (21.1451, 57.3243) (20.9969, 57.0674) knots 0 0 0 1 2 2 2
  spline S80 degree 2 poles (20.9969, 57.0674) (20.8487, 56.8006) (20.4189, 56.277) (20.1818, 56.0251) knots 0 0 0 1 2 2 2
  spline S81 degree 2 poles (20.1818, 56.0251) (19.7965, 55.6051) (18.853, 54.7061) (18.5714, 54.4442) knots 0 0 0 1 2 2 2
  line L152 (18.5714, 54.4442) -> (21.565, 54.4442)
  line L153 (21.565, 54.4442) -> (21.565, 53.7378)
  line L154 (26.1395, 53.7378) -> (22.3801, 53.7378)
  line L155 (22.3801, 53.7378) -> (22.3801, 54.6023)
  spline S82 degree 2 poles (22.3801, 54.6023) (22.7852, 54.9827) (23.5065, 55.6891) (23.8523, 56.0695) knots 0 0 0 1 2 2 2
  spline S83 degree 2 poles (23.8523, 56.0695) (24.5488, 56.8352) (25.0576, 57.7541) (25.0576, 58.2431) knots 0 0 0 1 2 2 2
  spline S84 degree 2 poles (25.0576, 58.2431) (25.0576, 58.5) (24.8996, 58.8853) (24.7563, 59.0088) knots 0 0 0 1 2 2 2
  spline S85 degree 2 poles (24.7563, 59.0088) (24.613, 59.1323) (24.2376, 59.2558) (24.0103, 59.2558) knots 0 0 0 1 2 2 2
  spline S86 degree 2 poles (24.0103, 59.2558) (23.793, 59.2558) (23.3484, 59.1472) (23.1458, 59.0632) knots 0 0 0 1 2 2 2
  spline S87 degree 2 poles (23.1458, 59.0632) (22.9729, 58.994) (22.6518, 58.7964) (22.553, 58.7272) knots 0 0 0 1 2 2 2
  line L156 (22.553, 58.7272) -> (22.5086, 58.7272)
  line L157 (22.5086, 58.7272) -> (22.5086, 59.5967)
  spline S88 degree 2 poles (22.5086, 59.5967) (22.7605, 59.7202) (23.6645, 59.9623) (24.0696, 59.9623) knots 0 0 0 1 2 2 2
  spline S89 degree 2 poles (24.0696, 59.9623) (24.9243, 59.9623) (25.8876, 59.0582) (25.8876, 58.2876) knots 0 0 0 1 2 2 2
  spline S90 degree 2 poles (25.8876, 58.2876) (25.8876, 57.927) (25.7196, 57.3243) (25.5714, 57.0674) knots 0 0 0 1 2 2 2
  spline S91 degree 2 poles (25.5714, 57.0674) (25.4232, 56.8006) (24.9934, 56.277) (24.7563, 56.0251) knots 0 0 0 1 2 2 2
  spline S92 degree 2 poles (24.7563, 56.0251) (24.371, 55.6051) (23.4274, 54.7061) (23.1458, 54.4442) knots 0 0 0 1 2 2 2
  line L158 (23.1458, 54.4442) -> (26.1395, 54.4442)
  line L159 (26.1395, 54.4442) -> (26.1395, 53.7378)
  line L160 (29.4888, 60.1055) -> (27.1028, 52.4139)
  line L161 (27.1028, 52.4139) -> (26.4112, 52.4139)
  line L162 (26.4112, 52.4139) -> (28.7874, 60.1055)
  line L163 (28.7874, 60.1055) -> (29.4888, 60.1055)
  line L164 (33.9201, 53.7378) -> (30.1607, 53.7378)
  line L165 (30.1607, 53.7378) -> (30.1607, 54.6023)
  spline S93 degree 2 poles (30.1607, 54.6023) (30.5658, 54.9827) (31.287, 55.6891) (31.6328, 56.0695) knots 0 0 0 1 2 2 2
  spline S94 degree 2 poles (31.6328, 56.0695) (32.3294, 56.8352) (32.8382, 57.7541) (32.8382, 58.2431) knots 0 0 0 1 2 2 2
  spline S95 degree 2 poles (32.8382, 58.2431) (32.8382, 58.5) (32.6801, 58.8853) (32.5368, 59.0088) knots 0 0 0 1 2 2 2
  spline S96 degree 2 poles (32.5368, 59.0088) (32.3936, 59.1323) (32.0181, 59.2558) (31.7909, 59.2558) knots 0 0 0 1 2 2 2
  spline S97 degree 2 poles (31.7909, 59.2558) (31.5735, 59.2558) (31.1289, 59.1472) (30.9264, 59.0632) knots 0 0 0 1 2 2 2
  spline S98 degree 2 poles (30.9264, 59.0632) (30.7535, 58.994) (30.4324, 58.7964) (30.3336, 58.7272) knots 0 0 0 1 2 2 2
  line L166 (30.3336, 58.7272) -> (30.2891, 58.7272)
  line L167 (30.2891, 58.7272) -> (30.2891, 59.5967)
  spline S99 degree 2 poles (30.2891, 59.5967) (30.5411, 59.7202) (31.4451, 59.9623) (31.8502, 59.9623) knots 0 0 0 1 2 2 2
  spline S100 degree 2 poles (31.8502, 59.9623) (32.7048, 59.9623) (33.6681, 59.0582) (33.6681, 58.2876) knots 0 0 0 1 2 2 2
  spline S101 degree 2 poles (33.6681, 58.2876) (33.6681, 57.927) (33.5002, 57.3243) (33.3519, 57.0674) knots 0 0 0 1 2 2 2
  spline S102 degree 2 poles (33.3519, 57.0674) (33.2037, 56.8006) (32.774, 56.277) (32.5368, 56.0251) knots 0 0 0 1 2 2 2
  spline S103 degree 2 poles (32.5368, 56.0251) (32.1515, 55.6051) (31.208, 54.7061) (30.9264, 54.4442) knots 0 0 0 1 2 2 2
  line L168 (30.9264, 54.4442) -> (33.9201, 54.4442)
  line L169 (33.9201, 54.4442) -> (33.9201, 53.7378)
  spline S104 degree 2 poles (38.4303, 55.6743) (38.4303, 55.2346) (38.1487, 54.4838) (37.8918, 54.2071) knots 0 0 0 1 2 2 2
  spline S105 degree 2 poles (37.8918, 54.2071) (37.635, 53.9305) (36.8693, 53.6094) (36.395, 53.6094) knots 0 0 0 1 2 2 2
  spline S106 degree 2 poles (36.395, 53.6094) (35.9603, 53.6094) (35.1106, 53.802) (34.7994, 53.9552) knots 0 0 0 1 2 2 2
  line L170 (34.7994, 53.9552) -> (34.7994, 54.8197)
  line L171 (34.7994, 54.8197) -> (34.8587, 54.8197)
  spline S107 degree 2 poles (34.8587, 54.8197) (34.9525, 54.7505) (35.3033, 54.5727) (35.5157, 54.4936) knots 0 0 0 1 2 2 2
  spline S108 degree 2 poles (35.5157, 54.4936) (35.7577, 54.4097) (36.1579, 54.3158) (36.4098, 54.3158) knots 0 0 0 1 2 2 2
  spline S109 degree 2 poles (36.4098, 54.3158) (36.6568, 54.3158) (37.1212, 54.4936) (37.2892, 54.6863) knots 0 0 0 1 2 2 2
  spline S110 degree 2 poles (37.2892, 54.6863) (37.4423, 54.8691) (37.6004, 55.3532) (37.6004, 55.6792) knots 0 0 0 1 2 2 2
  spline S111 degree 2 poles (37.6004, 55.6792) (37.6004, 56.0053) (37.4225, 56.4203) (37.2546, 56.5586) knots 0 0 0 1 2 2 2
  spline S112 degree 2 poles (37.2546, 56.5586) (37.0817, 56.7117) (36.5679, 56.8402) (36.2567, 56.8402) knots 0 0 0 1 2 2 2
  spline S113 degree 2 poles (36.2567, 56.8402) (35.9208, 56.8402) (35.2539, 56.7364) (35.0513, 56.692) knots 0 0 0 1 2 2 2
  line L172 (35.0513, 56.692) -> (35.0513, 59.8338)
  line L173 (35.0513, 59.8338) -> (38.3957, 59.8338)
  line L174 (38.3957, 59.8338) -> (38.3957, 59.1175)
  line L175 (38.3957, 59.1175) -> (35.8368, 59.1175)
  line L176 (35.8368, 59.1175) -> (35.8368, 57.4922)
  spline S114 degree 2 poles (35.8368, 57.4922) (35.985, 57.512) (36.2715, 57.5268) (36.3901, 57.5268) knots 0 0 0 1 2 2 2
  spline S115 degree 2 poles (36.3901, 57.5268) (36.8594, 57.5268) (37.5065, 57.3737) (37.8029, 57.1464) knots 0 0 0 1 2 2 2
  spline S116 degree 2 poles (37.8029, 57.1464) (38.1043, 56.9192) (38.4303, 56.2276) (38.4303, 55.6743) knots 0 0 0 1 2 2 2
  point P0 (-108.185, -10)
  constraints: 2 other
emboss "LABEL" sketch "Sketch30" operation cut depth 1 direction (-1, 0, 0)
sketch "Sketch31" plane through (0, 0, 0) normal (1, 0, 0) x (0, 1, 0)
  line L0 (0, -129.2475) -> (0, 135) projected
  line L1 (0, -112.5) -> (2.8, -112.5)
  line L2 (2.8, -112.5) -> (2.8, -115.5)
  line L3 (2.8, -115.5) -> (0, -115.5)
  line L4 (0, -115.5) -> (0, -112.5)
  line L5 (-22.1, 0) -> (132.6, 0) projected
  point P0 (0, 0)
  point P1 (0, -114)
  dimension "d211" = 2.8
  dimension "d212" = 3
  dimension "d213" = 114
  constraints: 8 end point, 2 parallel, 1 horizontal, 1 midpoint, 1 perpendicular, 1 point on line
  measures "d211" distance of L2.end L3.end
  measures "d212" distance of L1.end L2.end
  measures "d213" distance of point (0, 0) point (0, -114)
revolve "Seal Groove" cut sketch "Sketch31" angle 360 about axis through (0, -10, 0) along (0, 1, 0)
ref_plane "Work Plane3" through (0, 81.5, 0) normal (0, -1, 0) x (-0.5, 0, -0.8660254)
ref_plane "Work Plane4" through (0, 81.5, 0) normal (0, -1, 0) x (-0.5, 0, 0.8660254)
body "Solid1"
